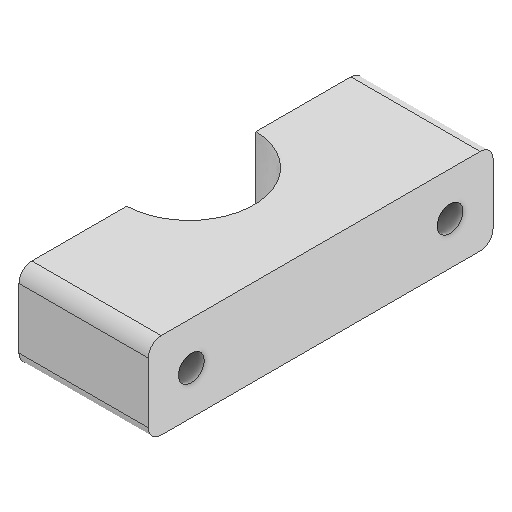
# Autodesk Inventor part: 3DP_ASA_Balcony_Mounting_Clamp_Front
Saved by Autodesk Inventor 2026.1 (Build 301233000, 233)
## iProperties
Created: 2025-06-22
Part Number: 3DP_ASA_Balcony_Mounting_Clamp_Front
Material: Generic
Document SubType Name: Modeling
Designer: User
Density: 1 g/cm^3
Appearance: Default
Author: User
Autodesk Inventor part; units mm, degrees
ref_plane "YZ Plane" through (0, 0, 0) normal (1, 0, 0) x (0, 1, 0)
ref_plane "XZ Plane" through (0, 0, 0) normal (0, 1, 0) x (-1, 0, 0)
ref_plane "XY Plane" through (0, 0, 0) normal (0, 0, 1) x (1, 0, 0)
sketch "Sketch1" plane through (0, 0, 0) normal (0, 1, 0) x (-1, 0, 0)
  line L0 (-15, 40) -> (15, 40)
  line L1 (15, 40) -> (15, -40)
  line L2 (15, -40) -> (-15, -40)
  line L3 (-15, -40) -> (-15, 40)
  arc A0 (15, 14.9917) -> (15, -14.9917) centre (15.5, 0) ccw
  point P0 (0, 0)
  dimension "d0" = 80
  dimension "d1" = 30
  dimension "d2" = 40
  dimension "d3" = 15
  dimension "d4" = 30
  dimension "d22" = 0.5
  constraints: 8 end point, 2 parallel, 2 point on circle, 2 point on line, 1 centre point, 1 horizontal, 1 perpendicular
  measures "d0" distance between parallel lines of L2 L0
  measures "d1" distance between parallel lines of L3 L1
  measures "d2" distance from line of point (0, 0) L0
  measures "d3" distance from line of L1 point (0, 0)
  measures "d4" diameter of A0
  measures "d22" distance from line of L1 A0.centre
extrude "Extrusion1" add sketch "Sketch1" along normal blind 20 contours L0 L1 A0 L2 L3
sketch "Sketch2" plane through (15, 0, 40) normal (1, 0, 0) x (0, 0, -1)
  line L0 (0, 0) -> (80, 0) projected
  line L1 (80, 0) -> (80, 20) projected
  line L2 (0, 20) -> (80, 20) projected
  line L3 (0, 0) -> (0, 20) projected
  point P0 (40, 0)
  point P1 (10, 10)
  point P2 (70, 10)
  dimension "d8" = 10
  dimension "d9" = 10
  dimension "d10" = 10
  dimension "d11" = 10
  measures "d8" distance from line of L3 point (10, 10)
  measures "d9" distance from line of L1 point (70, 10)
  measures "d10" distance from line of L2 point (10, 10)
  measures "d11" distance from line of L2 point (70, 10)
hole "Hole1" at (15, 10, 30) at (15, 10, -30) direction (-1, 0, 0) diameter 6 end through all
fillet "Fillet1" radius 3 4 edges at (0, 20, -40) (0, 20, 40) (0, 0, 40) (0, 0, -40)
equation "\"d2\" = 0.5 * d0"
equation "\"d3\" = 0.5 * d1"
equation "\"d9\" = d8"
body "Solid1"
